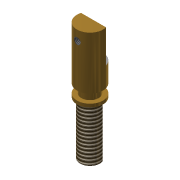
# Autodesk Inventor part: rod
Saved by Autodesk Inventor 2015 (Build 190159000, 159)
## iProperties
Created: 2015-10-28
Part Number: rod
Material: Generic
Document SubType Name: Modeling
Designer: jad211
Density: 1 g/cm^3
Appearance: Default
Author: jad211
Autodesk Inventor part; units mm, degrees
ref_plane "YZ Plane" through (0, 0, 0) normal (1, 0, 0) x (0, 1, 0)
ref_plane "XZ Plane" through (0, 0, 0) normal (0, 1, 0) x (-1, 0, 0)
ref_plane "XY Plane" through (0, 0, 0) normal (0, 0, 1) x (1, 0, 0)
sketch "Sketch1" plane through (0, 0, 0) normal (0, 1, 0) x (-1, 0, 0)
  line L0 (0, 0) -> (-2.8001, 0)
  line L1 (-2.8001, 0) -> (-3.937, 0)
  line L2 (-3.937, 0) -> (-3.937, -16)
  line L3 (-3.937, -16) -> (-2.6225, -16)
  line L4 (-2.6225, -16) -> (-2.6225, -18.6416)
  line L5 (-2.6225, -18.6416) -> (-3.937, -18.6416)
  line L6 (-3.937, -18.6416) -> (-3.937, -19.6416)
  line L7 (-2.8001, 0) -> (0, 0)
  line L8 (-2.8001, 0) -> (0, 0)
  line L9 (-3.937, -19.6416) -> (-3, -19.6416)
  line L10 (-3, -19.6416) -> (-3, -35.6416)
  line L11 (-3, -35.6416) -> (0, -35.6416)
  line L12 (0, -35.6416) -> (0, 0)
  dimension "d1" = 0
  dimension "d2" = 16
  dimension "d3" = 2.6416
  dimension "d6" = 3.937
  dimension "d8" = 3
  dimension "d13" = 1
  dimension "d29" = 2.6225
  dimension "d30" = 16
  constraints: 26 end point, 7 perpendicular, 3 horizontal, 2 point on line, 1 collinear
  measures "d1" distance of L0.end L1.start
  measures "d2" distance of L1.end L2.end
  measures "d3" distance of L3.end L4.end
  measures "d6" distance between parallel lines of L6 L12
  measures "d8" distance of L10.end L11.end
  measures "d13" distance of L5.end L6.end
  measures "d29" distance from line of L12 L3.end
  measures "d30" distance of L9.end L10.end
revolve "Revolution1" add sketch "Sketch1" angle 360 about axis through (0, 0, -35.6416) along (0, 0, 1)
thread "Thread1" size "M6x1" class "6g" standard "ANSI Metric M Profile" full length
sketch "Sketch3" plane through (0, 0, 0) normal (0, 0, 1) x (1, 0, 0)
  circle A0 centre (0, 0) radius 3.937 projected
  line L0 (-3.033, -2.5101) -> (3.033, -2.5101)
  line L1 (-3.7908, 1.063) -> (3.7908, 1.063)
  arc A1 (3.033, -2.5101) -> (3.7908, 1.063) centre (0, 0) ccw
  arc A2 (-3.7908, 1.063) -> (-3.033, -2.5101) centre (0, 0) ccw
  point P0 (0, 0)
  dimension "d36" = 5
  constraints: 8 point on circle, 4 end point, 2 centre point, 1 coincident, 1 horizontal, 1 parallel
extrude "Extrusion1" cut sketch "Sketch3" against normal blind 10 contours L1 A0
sketch "Sketch4" plane through (-3.7908, 1.063, 0) normal (0, 1, 0) x (1, 0, 0)
  circle A0 centre (3.7908, 3) radius 1
  point P0 (3.7908, 0)
  dimension "d23" = 2
  dimension "d24" = 3
  constraints: 1 centre point
  measures "d23" diameter of A0
  measures "d24" distance of point (3.791, 0) A0.centre
extrude "Extrusion2" cut sketch "Sketch4" against normal blind 10
thread "Thread2" size "M2x0.4" class "6H" standard "ANSI Metric M Profile" full length
sketch "Sketch5" plane through (0, 0, -35.6416) normal (0, 0, -1) x (-1, 0, 0)
  circle A0 centre (0, 0) radius 3.937 projected
  line L0 (-3.7908, 1.063) -> (5.4234, 1.063)
  line L1 (5.4234, 1.063) -> (5.4234, 3.7958)
  line L2 (5.4234, 3.7958) -> (-3.7908, 3.7958)
  line L3 (-3.7908, 3.7958) -> (-3.7908, 1.063)
  point P0 (0, 0)
  dimension "d33" = 5
  constraints: 8 end point, 2 parallel, 1 horizontal, 1 perpendicular, 2 other
extrude "Extrusion3" cut sketch "Sketch5" against normal blind 16 contours L3 L2 A0 | A0 L2 L0 | A0 L2 L1 L0
body "Solid1"
